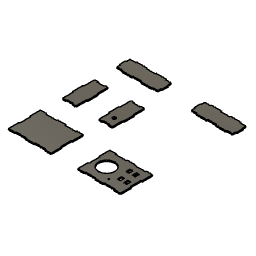
12.BOXパーツ (Autodesk Fusion 360 design; units mm, degrees)
Autodesk Fusion 360 part; units mm, degrees
sketch "スケッチ1" plane through (0, 0, 0) normal (0, 0, 1) x (1, 0, 0)
  line L0 (0, 0) -> (200, 0)
  line L1 (200, 0) -> (200, 150)
  line L2 (200, 150) -> (0, 150)
  line L3 (0, 150) -> (0, 0)
  line L4 (30, 150) -> (80, 150)
  line L5 (80, 150) -> (80, 146)
  line L6 (80, 146) -> (30, 146)
  line L7 (30, 146) -> (30, 150)
  line L8 (120, 150) -> (170, 150)
  line L9 (170, 150) -> (170, 146)
  line L10 (170, 146) -> (120, 146)
  line L11 (120, 146) -> (120, 150)
  line L12 (0, 50) -> (4, 50)
  line L13 (4, 50) -> (4, 100)
  line L14 (4, 100) -> (0, 100)
  line L15 (0, 100) -> (0, 50)
  line L16 (200, 100) -> (196, 100)
  line L17 (196, 100) -> (196, 50)
  line L18 (196, 50) -> (200, 50)
  line L19 (200, 50) -> (200, 100)
  line L20 (30, 0) -> (80, 0)
  line L21 (80, 0) -> (80, 4)
  line L22 (80, 4) -> (30, 4)
  line L23 (30, 4) -> (30, 0)
  line L24 (120, 0) -> (170, 0)
  line L25 (170, 0) -> (170, 4)
  line L26 (170, 4) -> (120, 4)
  line L27 (120, 4) -> (120, 0)
  line L28 (325, 100) -> (325, 50)
  line L29 (525, 150) -> (325, 150)
  line L30 (405, 146) -> (355, 146)
  line L31 (355, 146) -> (355, 150)
  line L32 (405, 4) -> (355, 4)
  line L33 (521, 100) -> (521, 50)
  line L34 (445, 4) -> (445, 0)
  line L35 (495, 146) -> (445, 146)
  line L36 (525, 100) -> (521, 100)
  line L37 (521, 50) -> (525, 50)
  line L38 (355, 0) -> (405, 0)
  line L39 (525, 0) -> (525, 150)
  line L40 (495, 0) -> (495, 4)
  line L41 (405, 0) -> (405, 4)
  line L42 (355, 4) -> (355, 0)
  line L43 (445, 146) -> (445, 150)
  line L44 (325, 0) -> (525, 0)
  line L45 (325, 50) -> (329, 50)
  line L46 (525, 50) -> (525, 100)
  line L47 (329, 100) -> (325, 100)
  line L48 (325, 150) -> (325, 0)
  line L49 (445, 150) -> (495, 150)
  line L50 (495, 4) -> (445, 4)
  line L51 (329, 50) -> (329, 100)
  line L52 (495, 150) -> (495, 146)
  line L53 (355, 150) -> (405, 150)
  line L54 (405, 150) -> (405, 146)
  line L55 (445, 0) -> (495, 0)
  line L56 (0, 250) -> (70, 250)
  line L57 (70, 250) -> (70, 400)
  line L58 (70, 400) -> (0, 400)
  line L59 (0, 400) -> (0, 250)
  line L60 (0, 400) -> (4, 400)
  line L61 (4, 400) -> (4, 350)
  line L62 (4, 350) -> (0, 350)
  line L63 (0, 350) -> (0, 400)
  line L64 (0, 250) -> (4, 250)
  line L65 (4, 250) -> (4, 300)
  line L66 (4, 300) -> (0, 300)
  line L67 (0, 300) -> (0, 250)
  line L68 (70, 400) -> (66, 400)
  line L69 (66, 400) -> (66, 350)
  line L70 (66, 350) -> (70, 350)
  line L71 (70, 350) -> (70, 400)
  line L72 (70, 250) -> (66, 250)
  line L73 (66, 250) -> (66, 300)
  line L74 (66, 300) -> (70, 300)
  line L75 (70, 300) -> (70, 250)
  line L76 (20, 400) -> (50, 400)
  line L77 (50, 400) -> (50, 396)
  line L78 (50, 396) -> (20, 396)
  line L79 (20, 396) -> (20, 400)
  line L80 (20, 250) -> (50, 250)
  line L81 (50, 250) -> (50, 254)
  line L82 (50, 254) -> (20, 254)
  line L83 (20, 254) -> (20, 250)
  line L84 (220, 396) -> (190, 396)
  line L85 (240, 250) -> (240, 400)
  line L86 (236, 350) -> (240, 350)
  line L87 (170, 400) -> (174, 400)
  line L88 (240, 400) -> (236, 400)
  line L89 (174, 250) -> (174, 300)
  line L90 (174, 350) -> (170, 350)
  line L91 (240, 350) -> (240, 400)
  line L92 (236, 250) -> (236, 300)
  line L93 (190, 254) -> (190, 250)
  line L94 (170, 250) -> (240, 250)
  line L95 (240, 300) -> (240, 250)
  line L96 (220, 400) -> (220, 396)
  line L97 (190, 250) -> (220, 250)
  line L98 (240, 250) -> (236, 250)
  line L99 (170, 300) -> (170, 250)
  line L100 (220, 254) -> (190, 254)
  line L101 (170, 250) -> (174, 250)
  line L102 (174, 300) -> (170, 300)
  line L103 (170, 350) -> (170, 400)
  line L104 (174, 400) -> (174, 350)
  line L105 (190, 396) -> (190, 400)
  line L106 (170, 400) -> (170, 250)
  line L107 (236, 300) -> (240, 300)
  line L108 (236, 400) -> (236, 350)
  line L109 (220, 250) -> (220, 254)
  line L110 (240, 400) -> (170, 400)
  line L111 (190, 400) -> (220, 400)
  line L112 (0, 500) -> (200, 500)
  line L113 (200, 500) -> (200, 570)
  line L114 (200, 570) -> (0, 570)
  line L115 (0, 570) -> (0, 500)
  line L116 (0, 570) -> (4, 570)
  line L117 (4, 570) -> (4, 550)
  line L118 (4, 550) -> (0, 550)
  line L119 (0, 550) -> (0, 570)
  line L120 (0, 500) -> (4, 500)
  line L121 (4, 500) -> (4, 520)
  line L122 (4, 520) -> (0, 520)
  line L123 (0, 520) -> (0, 500)
  line L124 (200, 570) -> (196, 570)
  line L125 (196, 570) -> (196, 550)
  line L126 (196, 550) -> (200, 550)
  line L127 (200, 550) -> (200, 570)
  line L128 (200, 500) -> (196, 500)
  line L129 (196, 500) -> (196, 520)
  line L130 (196, 520) -> (200, 520)
  line L131 (200, 520) -> (200, 500)
  line L132 (0, 570) -> (30, 570)
  line L133 (30, 570) -> (30, 566)
  line L134 (30, 566) -> (0, 566)
  line L135 (0, 566) -> (0, 570)
  line L136 (80, 570) -> (120, 570)
  line L137 (120, 570) -> (120, 566)
  line L138 (120, 566) -> (80, 566)
  line L139 (80, 566) -> (80, 570)
  line L140 (170, 570) -> (200, 570)
  line L141 (200, 570) -> (200, 566)
  line L142 (200, 566) -> (170, 566)
  line L143 (170, 566) -> (170, 570)
  line L144 (0, 500) -> (30, 500)
  line L145 (30, 500) -> (30, 504)
  line L146 (30, 504) -> (0, 504)
  line L147 (0, 504) -> (0, 500)
  line L148 (200, 500) -> (170, 500)
  line L149 (170, 500) -> (170, 504)
  line L150 (170, 504) -> (200, 504)
  line L151 (200, 504) -> (200, 500)
  line L152 (80, 500) -> (120, 500)
  line L153 (120, 500) -> (120, 504)
  line L154 (120, 504) -> (80, 504)
  line L155 (80, 504) -> (80, 500)
  line L156 (350, 570) -> (350, 500)
  line L157 (350, 550) -> (350, 570)
  line L158 (350, 504) -> (350, 500)
  line L159 (350, 566) -> (350, 570)
  line L160 (350, 570) -> (380, 570)
  line L161 (354, 550) -> (350, 550)
  line L162 (380, 500) -> (380, 504)
  line L163 (354, 520) -> (350, 520)
  line L164 (350, 500) -> (354, 500)
  line L165 (380, 504) -> (350, 504)
  line L166 (350, 520) -> (350, 500)
  line L167 (350, 500) -> (380, 500)
  line L168 (550, 520) -> (550, 500)
  line L169 (520, 504) -> (550, 504)
  line L170 (550, 550) -> (550, 570)
  line L171 (550, 570) -> (550, 566)
  line L172 (546, 570) -> (546, 550)
  line L173 (550, 504) -> (550, 500)
  line L174 (546, 550) -> (550, 550)
  line L175 (550, 566) -> (520, 566)
  line L176 (430, 570) -> (470, 570)
  line L177 (470, 500) -> (470, 504)
  line L178 (380, 566) -> (350, 566)
  line L179 (430, 566) -> (430, 570)
  line L180 (350, 570) -> (354, 570)
  line L181 (380, 570) -> (380, 566)
  line L182 (354, 500) -> (354, 520)
  line L183 (430, 504) -> (430, 500)
  line L184 (550, 500) -> (550, 570)
  line L185 (354, 570) -> (354, 550)
  line L186 (550, 570) -> (546, 570)
  line L187 (546, 520) -> (550, 520)
  line L188 (470, 570) -> (470, 566)
  line L189 (430, 500) -> (470, 500)
  line L190 (520, 500) -> (520, 504)
  line L191 (350, 500) -> (550, 500)
  line L192 (470, 566) -> (430, 566)
  line L193 (470, 504) -> (430, 504)
  line L194 (550, 500) -> (520, 500)
  line L195 (546, 500) -> (546, 520)
  line L196 (520, 566) -> (520, 570)
  line L197 (550, 570) -> (350, 570)
  line L198 (550, 500) -> (546, 500)
  line L199 (520, 570) -> (550, 570)
  circle A0 centre (205, 290) radius 7.5
  circle A1 centre (385, 75) radius 38
  line L200 (450, 120) -> (463, 120)
  line L201 (463, 120) -> (463, 101)
  line L202 (463, 101) -> (450, 101)
  line L203 (450, 101) -> (450, 120)
  line L204 (480, 120) -> (493, 120)
  line L205 (493, 120) -> (493, 101)
  line L206 (480, 101) -> (480, 120)
  line L207 (493, 101) -> (480, 101)
  line L208 (490, 70) -> (503, 70)
  line L209 (460, 70) -> (473, 70)
  line L210 (503, 70) -> (503, 51)
  line L211 (460, 51) -> (460, 70)
  line L212 (503, 51) -> (490, 51)
  line L213 (490, 51) -> (490, 70)
  line L214 (473, 70) -> (473, 51)
  line L215 (473, 51) -> (460, 51)
  circle A2 centre (440, 30) radius 3.5
  point P0 (325, 0)
  dimension "d2" = 200
  dimension "d3" = 150
  dimension "d4" = 4
  dimension "d5" = 4
  dimension "d6" = 4
  dimension "d7" = 4
  dimension "d8" = 4
  dimension "d9" = 50
  dimension "d10" = 4
  dimension "d11" = 200
  dimension "d12" = 150
  dimension "d13" = 4
  dimension "d14" = 4
  dimension "d15" = 4
  dimension "d16" = 4
  dimension "d17" = 4
  dimension "d18" = 50
  dimension "d19" = 4
  dimension "d20" = 70
  dimension "d21" = 150
  dimension "d22" = 4
  dimension "d23" = 4
  dimension "d24" = 4
  dimension "d25" = 4
  dimension "d26" = 30
  dimension "d27" = 4
  dimension "d28" = 4
  dimension "d29" = 70
  dimension "d30" = 150
  dimension "d31" = 4
  dimension "d32" = 4
  dimension "d33" = 4
  dimension "d34" = 4
  dimension "d35" = 30
  dimension "d36" = 4
  dimension "d37" = 4
  dimension "d38" = 200
  dimension "d39" = 70
  dimension "d40" = 4
  dimension "d41" = 4
  dimension "d42" = 4
  dimension "d43" = 4
  dimension "d44" = 4
  dimension "d45" = 4
  dimension "d46" = 4
  dimension "d47" = 4
  dimension "d48" = 4
  dimension "d49" = 4
  dimension "d50" = 200
  dimension "d51" = 70
  dimension "d52" = 4
  dimension "d53" = 4
  dimension "d54" = 4
  dimension "d55" = 4
  dimension "d56" = 4
  dimension "d57" = 4
  dimension "d58" = 4
  dimension "d59" = 4
  dimension "d60" = 4
  dimension "d61" = 4
  dimension "d62" = 15
  dimension "d63" = 76
  dimension "d64" = 13
  dimension "d65" = 19
  dimension "d66" = 13
  dimension "d67" = 19
  dimension "d68" = 13
  dimension "d69" = 19
  dimension "d70" = 13
  dimension "d71" = 19
  dimension "d72" = 7
  constraint horizontal L0
  constraint vertical L1
  constraint horizontal L2
  constraint vertical L3
  constraint coincident L0.start L3.end
  constraint horizontal L4
  constraint vertical L5
  constraint horizontal L6
  constraint vertical L7
  constraint coincident L2 L4.start
  constraint horizontal L8
  constraint vertical L9
  constraint horizontal L10
  constraint vertical L11
  constraint coincident L2 L8.start
  constraint horizontal L12
  constraint vertical L13
  constraint horizontal L14
  constraint vertical L15
  constraint coincident L3 L12.start
  constraint horizontal L16
  constraint vertical L17
  constraint horizontal L18
  constraint vertical L19
  constraint coincident L1 L16.start
  constraint horizontal L20
  constraint vertical L21
  constraint horizontal L22
  constraint vertical L23
  constraint coincident L0 L20.start
  constraint horizontal L24
  constraint vertical L25
  constraint horizontal L26
  constraint vertical L27
  constraint coincident L0 L24.start
  constraint horizontal L44
  constraint vertical L39
  constraint horizontal L29
  constraint vertical L48
  constraint coincident P0 L44.start
  constraint horizontal L53
  constraint vertical L54
  constraint horizontal L30
  constraint vertical L31
  constraint coincident L31.end L29
  constraint horizontal L49
  constraint vertical L52
  constraint horizontal L35
  constraint vertical L43
  constraint coincident L43.end L29
  constraint horizontal L45
  constraint vertical L51
  constraint horizontal L47
  constraint vertical L28
  constraint coincident L28.end L48
  constraint horizontal L36
  constraint vertical L33
  constraint horizontal L37
  constraint vertical L46
  constraint coincident L36.start L39
  constraint horizontal L38
  constraint vertical L41
  constraint horizontal L32
  constraint vertical L42
  constraint coincident L38.start L44
  constraint horizontal L55
  constraint vertical L40
  constraint horizontal L50
  constraint vertical L34
  constraint coincident L34.end L44
  constraint horizontal L56
  constraint vertical L57
  constraint horizontal L58
  constraint vertical L59
  constraint horizontal L60
  constraint vertical L61
  constraint horizontal L62
  constraint vertical L63
  constraint horizontal L64
  constraint vertical L65
  constraint horizontal L66
  constraint vertical L67
  constraint horizontal L68
  constraint vertical L69
  constraint horizontal L70
  constraint vertical L71
  constraint horizontal L72
  constraint vertical L73
  constraint horizontal L74
  constraint vertical L75
  constraint horizontal L76
  constraint vertical L77
  constraint horizontal L78
  constraint vertical L79
  constraint coincident L58 L76.start
  constraint horizontal L80
  constraint vertical L81
  constraint horizontal L82
  constraint vertical L83
  constraint coincident L56 L80.start
  constraint horizontal L94
  constraint vertical L85
  constraint horizontal L110
  constraint vertical L106
  constraint horizontal L87
  constraint vertical L104
  constraint horizontal L90
  constraint vertical L103
  constraint horizontal L101
  constraint vertical L89
  constraint horizontal L102
  constraint vertical L99
  constraint horizontal L88
  constraint vertical L108
  constraint horizontal L86
  constraint vertical L91
  constraint horizontal L98
  constraint vertical L92
  constraint horizontal L107
  constraint vertical L95
  constraint horizontal L111
  constraint vertical L96
  constraint horizontal L84
  constraint vertical L105
  constraint coincident L105.end L110
  constraint horizontal L97
  constraint vertical L109
  constraint horizontal L100
  constraint vertical L93
  constraint coincident L93.end L94
  constraint horizontal L112
  constraint vertical L113
  constraint horizontal L114
  constraint vertical L115
  constraint horizontal L116
  constraint vertical L117
  constraint horizontal L118
  constraint vertical L119
  constraint horizontal L120
  constraint vertical L121
  constraint horizontal L122
  constraint vertical L123
  constraint horizontal L124
  constraint vertical L125
  constraint horizontal L126
  constraint vertical L127
  constraint horizontal L128
  constraint vertical L129
  constraint horizontal L130
  constraint vertical L131
  constraint horizontal L132
  constraint vertical L133
  constraint horizontal L134
  constraint vertical L135
  constraint horizontal L136
  constraint vertical L137
  constraint horizontal L138
  constraint vertical L139
  constraint coincident L114 L136.start
  constraint horizontal L140
  constraint vertical L141
  constraint horizontal L142
  constraint vertical L143
  constraint coincident L114 L140.start
  constraint horizontal L144
  constraint vertical L145
  constraint horizontal L146
  constraint vertical L147
  constraint horizontal L148
  constraint vertical L149
  constraint horizontal L150
  constraint vertical L151
  constraint horizontal L152
  constraint vertical L153
  constraint horizontal L154
  constraint vertical L155
  constraint coincident L112 L152.start
  constraint horizontal L191
  constraint vertical L184
  constraint horizontal L197
  constraint vertical L156
  constraint horizontal L180
  constraint vertical L185
  constraint horizontal L161
  constraint vertical L157
  constraint horizontal L164
  constraint vertical L182
  constraint horizontal L163
  constraint vertical L166
  constraint horizontal L186
  constraint vertical L172
  constraint horizontal L174
  constraint vertical L170
  constraint horizontal L198
  constraint vertical L195
  constraint horizontal L187
  constraint vertical L168
  constraint horizontal L160
  constraint vertical L181
  constraint horizontal L178
  constraint vertical L159
  constraint horizontal L176
  constraint vertical L188
  constraint horizontal L192
  constraint vertical L179
  constraint coincident L176.start L197
  constraint horizontal L199
  constraint vertical L171
  constraint horizontal L175
  constraint vertical L196
  constraint coincident L196.end L197
  constraint horizontal L167
  constraint vertical L162
  constraint horizontal L165
  constraint vertical L158
  constraint horizontal L194
  constraint vertical L190
  constraint horizontal L169
  constraint vertical L173
  constraint horizontal L189
  constraint vertical L177
  constraint horizontal L193
  constraint vertical L183
  constraint coincident L183.end L191
  constraint horizontal L200
  constraint vertical L201
  constraint horizontal L202
  constraint vertical L203
  constraint horizontal L204
  constraint vertical L205
  constraint horizontal L207
  constraint vertical L206
  constraint horizontal L209
  constraint vertical L214
  constraint horizontal L215
  constraint vertical L211
  constraint horizontal L208
  constraint vertical L210
  constraint horizontal L212
  constraint vertical L213
  measures "d2" distance of L0.start L0.end
  measures "d3" distance of L0.start L2.end
  measures "d4" distance of L4.start L6.end
  measures "d5" distance of L8.start L10.end
  measures "d6" distance of L12.start L12.end
  measures "d7" distance of L16.start L16.end
  measures "d8" distance of L20.start L22.end
  measures "d9" distance of L24.start L24.end
  measures "d10" distance of L24.start L26.end
  measures "d11" distance of P0 L39.start
  measures "d12" distance of P0 L29.end
  measures "d13" distance of L31.end L30.end
  measures "d14" distance of L43.end L35.end
  measures "d15" distance of L28.end L45.end
  measures "d16" distance of L36.start L33.start
  measures "d17" distance of L32.end L38.start
  measures "d18" distance of L40.start L34.end
  measures "d19" distance of L34.start L34.end
  measures "d20" distance of L56.start L56.end
  measures "d21" distance of L56.start L58.end
  measures "d22" distance of L58.end L60.end
  measures "d23" distance of L56.start L64.end
  measures "d24" distance of L57.end L68.end
  measures "d25" distance of L56.end L72.end
  measures "d26" distance of L76.start L76.end
  measures "d27" distance of L76.start L78.end
  measures "d28" distance of L80.start L82.end
  measures "d29" distance of L85.start L94.start
  measures "d30" distance of L87.start L94.start
  measures "d31" distance of L87.start L87.end
  measures "d32" distance of L94.start L89.start
  measures "d33" distance of L85.end L88.end
  measures "d34" distance of L85.start L92.start
  measures "d35" distance of L105.end L96.start
  measures "d36" distance of L84.end L105.end
  measures "d37" distance of L93.end L93.start
  measures "d38" distance of L112.start L112.end
  measures "d39" distance of L112.start L114.end
  measures "d40" distance of L114.end L116.end
  measures "d41" distance of L112.start L120.end
  measures "d42" distance of L113.end L124.end
  measures "d43" distance of L112.end L128.end
  measures "d44" distance of L114.end L134.end
  measures "d45" distance of L136.start L138.end
  measures "d46" distance of L140.start L142.end
  measures "d47" distance of L112.start L146.end
  measures "d48" distance of L112.end L150.end
  measures "d49" distance of L152.start L154.end
  measures "d50" distance of L168.end L156.end
  measures "d51" distance of L156.start L156.end
  measures "d52" distance of L156.start L180.end
  measures "d53" distance of L156.end L164.end
  measures "d54" distance of L170.end L172.start
  measures "d55" distance of L168.end L195.start
  measures "d56" distance of L156.start L159.start
  measures "d57" distance of L176.start L179.start
  measures "d58" distance of L175.end L196.end
  measures "d59" distance of L156.end L158.start
  measures "d60" distance of L168.end L169.end
  measures "d61" distance of L183.end L183.start
  measures "d62" diameter of A0
  measures "d63" diameter of A1
  measures "d64" distance of L200.start L200.end
  measures "d65" distance of L200.start L202.end
  measures "d66" distance of L204.start L204.end
  measures "d67" distance of L204.start L206.start
  measures "d68" distance of L209.start L209.end
  measures "d69" distance of L209.start L211.start
  measures "d70" distance of L208.end L208.start
  measures "d71" distance of L212.end L208.start
  measures "d72" diameter of A2
sketch "スケッチ2" plane through (0, 0, 0) normal (0, 0, 1) x (1, 0, 0)
extrude "押し出し1" add sketch "スケッチ1" along normal blind 5.5 contours L0 L1 L2 L3 L5 L6 L7 L9 L10 L11 L12 L13 L14 L16 L17 L18 L21 L22 L23 L25 L26 L27 | L29 L30 L31 L32 L33 L34 L35 L36 L37 L39 L40 L41 L42 L43 L44 L45 L47 L48 L50 L51 L52 L54 | L56 L57 L58 L59 L61 L62 L65 L66 L69 L70 L73 L74 L77 L78 L79 L81 L82 L83 | L84 L85 L86 L89 L90 L92 L93 L94 L96 L100 L102 L104 L105 L106 L107 L108 L109 L110 | L112 L113 L114 L115 L117 L118 L121 L122 L125 L126 L129 L130 L133 L134 L137 L138 L139 L142 L143 L145 L146 L149 L150 L153 L154 L155 | L156 L161 L162 L163 L165 L169 L172 L174 L175 L177 L178 L179 L181 L182 L183 L184 L185 L187 L188 L190 L191 L192 L193 L195 L196 L197 makes body 1 at (40, 284.6667, 0) makes body 2 at (46.6667, 545.3333, 0) makes body 3 at (54.6667, 66.6667, 0) makes body 4 at (204.8132, 332.493, 0) makes body 5 at (396.6667, 545.3333, 0) makes body 6 at (470.4482, 27.9895, 0)
